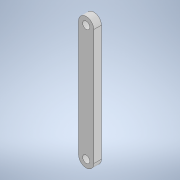
# Autodesk Inventor part: Linkage
Saved by Autodesk Inventor 2022 (Build 260153000, 153)
## iProperties
Created: 2022-04-03
Part Number: Linkage
Material: Generic
Document SubType Name: Modeling
Designer: Nick
Density: 1 g/cm^3
Appearance: Default
Author: Nick
Autodesk Inventor part; units mm, degrees
ref_plane "YZ Plane" through (0, 0, 0) normal (1, 0, 0) x (0, 1, 0)
ref_plane "XZ Plane" through (0, 0, 0) normal (0, 1, 0) x (-1, 0, 0)
ref_plane "XY Plane" through (0, 0, 0) normal (0, 0, 1) x (1, 0, 0)
sketch "Sketch1" plane through (0, 0, 0) normal (0, 0, 1) x (1, 0, 0)
  line L0 (0, 0) -> (6.35, 0)
  line L1 (6.35, 0) -> (6.35, 54.9181)
  line L2 (6.35, 54.9181) -> (0, 54.9181)
  line L3 (0, 54.9181) -> (0, 0)
  point P0 (3.175, 3.175)
  point P1 (3.175, 51.7431)
  point P2 (3.175, 0)
  dimension "d0" = 48.5681
  dimension "d1" = 3.175
  dimension "d2" = 3.175
  dimension "d3" = 6.35
  constraints: 8 end point, 2 parallel, 2 vertical alignment, 1 horizontal, 1 midpoint, 1 perpendicular
  measures "d0" distance of point (3.175, 51.743) point (3.175, 3.175)
  measures "d1" distance from line of L2 point (3.175, 51.743)
  measures "d2" distance from line of L0 point (3.175, 3.175)
  measures "d3" distance of L1.end L2.end
extrude "Extrusion1" add sketch "Sketch1" along normal blind 3.175
hole "Hole1" at (3.175, 3.175, 0) at (3.175, 51.7431, 0) direction (0, 0, 1) diameter 3 end through all
fillet "Fillet1" radius 3.175 4 edges at (6.35, 0, 1.5875) (0, 0, 1.5875) (0, 54.9181, 1.5875) (6.35, 54.9181, 1.5875)
body "Solid1"
